Autodesk Fusion 360 part; units mm, degrees
note: some values were not read from the file. Set by a fixed rule: the direction of a hole.
(part 4 of 8)
  spline S367 degree 3 poles (-140.5026, -58.4189) (-140.4982, -58.6928) (-140.4948, -58.9667) (-140.4926, -59.2407) knots 0 0 0 0 1 1 1 1
  spline S368 degree 3 poles (-140.4926, -59.2407) (-140.4892, -59.6344) (-140.4818, -60.028) (-140.4736, -60.4216) knots 0 0 0 0 1 1 1 1
  spline S369 degree 3 poles (-140.4736, -60.4216) (-140.4734, -60.5442) (-140.4732, -60.6668) (-140.473, -60.793) knots 0 0 0 0 1 1 1 1
  spline S370 degree 3 poles (-140.473, -60.793) (-140.4555, -61.482) (-140.4555, -61.482) (-140.0812, -62.0375) knots 0 0 0 0 1 1 1 1
  spline S371 degree 3 poles (-140.0812, -62.0375) (-139.5767, -62.271) (-139.3177, -62.2016) (-138.7893, -62.0358) knots 0 0 0 0 1 1 1 1
  spline S372 degree 3 poles (-138.7893, -62.0358) (-138.1237, -61.7626) (-138.1237, -61.7626) (-137.6781, -61.2421) knots 0 0 0 0 1 1 1 1
  spline S373 degree 3 poles (-137.6781, -61.2421) (-137.5109, -60.3536) (-137.5224, -59.4745) (-137.5293, -58.5731) knots 0 0 0 0 1 1 1 1
  spline S374 degree 3 poles (-137.5293, -58.5731) (-137.5272, -58.3243) (-137.5246, -58.0755) (-137.5215, -57.8268) knots 0 0 0 0 1 1 1 1
  spline S375 degree 3 poles (-137.5215, -57.8268) (-137.515, -57.2188) (-137.5154, -56.6113) (-137.5193, -56.0033) knots 0 0 0 0 1 1 1 1
  spline S376 degree 3 poles (-137.5193, -56.0033) (-137.205, -56.0033) (-136.8907, -56.0033) (-136.5668, -56.0033) knots 0 0 0 0 1 1 1 1
  spline S377 degree 3 poles (-136.5668, -56.0033) (-136.5668, -58.256) (-136.5668, -60.5086) (-136.5668, -62.8296) knots 0 0 0 0 1 1 1 1
  spline S378 degree 3 poles (-136.5668, -62.8296) (-136.8812, -62.8296) (-137.1955, -62.8296) (-137.5193, -62.8296) knots 0 0 0 0 1 1 1 1
  spline S379 degree 3 poles (-137.5193, -62.8296) (-137.5717, -62.6724) (-137.6241, -62.5152) (-137.6781, -62.3533) knots 0 0 0 0 1 1 1 1
  spline S380 degree 3 poles (-137.6781, -62.3533) (-137.8287, -62.4581) (-137.9793, -62.5629) (-138.1345, -62.6708) knots 0 0 0 0 1 1 1 1
  spline S381 degree 3 poles (-138.1345, -62.6708) (-138.8626, -63.0806) (-139.5601, -63.1684) (-140.3768, -62.9883) knots 0 0 0 0 1 1 1 1
  spline S382 degree 3 poles (-135.0686, -77.4941) (-135.9231, -76.9719) (-136.4768, -76.235) (-136.7944, -75.284) knots 0 0 0 0 1 1 1 1
  spline S383 degree 3 poles (-136.7944, -75.284) (-137.183, -73.601) (-137.2588, -71.5992) (-136.3684, -70.0626) knots 0 0 0 0 1 1 1 1
  spline S384 degree 3 poles (-136.3684, -70.0626) (-135.7688, -69.2218) (-135.1227, -68.6286) (-134.0696, -68.4212) knots 0 0 0 0 1 1 1 1
  spline S385 degree 3 poles (-134.0696, -68.4212) (-132.935, -68.3098) (-131.9094, -68.415) (-130.9659, -69.0878) knots 0 0 0 0 1 1 1 1
  spline S386 degree 3 poles (-130.9659, -69.0878) (-129.9714, -70.0009) (-129.6245, -71.1542) (-129.5471, -72.4674) knots 0 0 0 0 1 1 1 1
  spline S387 degree 3 poles (-129.5471, -72.4674) (-129.4973, -74.0526) (-129.5833, -75.5982) (-130.6162, -76.8833) knots 0 0 0 0 1 1 1 1
  spline S388 degree 3 poles (-130.6162, -76.8833) (-131.7464, -78.0045) (-133.6433, -78.1378) (-135.0686, -77.4941) knots 0 0 0 0 1 1 1 1
  spline S389 degree 3 poles (-131.3082, -76.1546) (-130.3984, -74.7293) (-130.3552, -73.0615) (-130.6435, -71.4318) knots 0 0 0 0 1 1 1 1
  spline S390 degree 3 poles (-130.6435, -71.4318) (-130.8576, -70.6183) (-131.2038, -69.9356) (-131.9296, -69.476) knots 0 0 0 0 1 1 1 1
  spline S391 degree 3 poles (-131.9296, -69.476) (-132.7297, -69.1221) (-133.5092, -69.0729) (-134.3443, -69.3383) knots 0 0 0 0 1 1 1 1
  spline S392 degree 3 poles (-134.3443, -69.3383) (-135.012, -69.7012) (-135.4666, -70.1853) (-135.7632, -70.8861) knots 0 0 0 0 1 1 1 1
  spline S393 degree 3 poles (-135.7632, -70.8861) (-136.1825, -72.4299) (-136.191, -74.42) (-135.4897, -75.87) knots 0 0 0 0 1 1 1 1
  spline S394 degree 3 poles (-135.4897, -75.87) (-135.1461, -76.3948) (-134.7368, -76.6827) (-134.1856, -76.9583) knots 0 0 0 0 1 1 1 1
  spline S395 degree 3 poles (-134.1856, -76.9583) (-132.9719, -77.0599) (-132.2031, -77.0231) (-131.3082, -76.1546) knots 0 0 0 0 1 1 1 1
  spline S396 degree 3 poles (-144.4448, -77.4842) (-145.1477, -76.7998) (-145.4309, -76.1732) (-145.4703, -75.1952) knots 0 0 0 0 1 1 1 1
  spline S397 degree 3 poles (-145.4703, -75.1952) (-145.4752, -74.783) (-145.4747, -74.3711) (-145.4723, -73.9588) knots 0 0 0 0 1 1 1 1
  spline S398 degree 3 poles (-145.4723, -73.9588) (-145.4721, -73.8084) (-145.4719, -73.658) (-145.4717, -73.5031) knots 0 0 0 0 1 1 1 1
  spline S399 degree 3 poles (-145.4717, -73.5031) (-145.4708, -73.0243) (-145.4688, -72.5456) (-145.4668, -72.0668) knots 0 0 0 0 1 1 1 1
  spline S400 degree 3 poles (-145.4668, -72.0668) (-145.466, -71.7416) (-145.4652, -71.4163) (-145.4646, -71.0911) knots 0 0 0 0 1 1 1 1
  spline S401 degree 3 poles (-145.4646, -71.0911) (-145.4628, -70.2952) (-145.4601, -69.4992) (-145.4568, -68.7033) knots 0 0 0 0 1 1 1 1
  spline S402 degree 3 poles (-145.4568, -68.7033) (-145.1425, -68.7033) (-144.8282, -68.7033) (-144.5043, -68.7033) knots 0 0 0 0 1 1 1 1
  spline S403 degree 3 poles (-144.5043, -68.7033) (-144.4996, -68.9747) (-144.4996, -68.9747) (-144.4948, -69.2515) knots 0 0 0 0 1 1 1 1
  spline S404 degree 3 poles (-144.4948, -69.2515) (-144.4827, -69.9273) (-144.4686, -70.603) (-144.454, -71.2787) knots 0 0 0 0 1 1 1 1
  spline S405 degree 3 poles (-144.454, -71.2787) (-144.4479, -71.5703) (-144.4424, -71.8619) (-144.4374, -72.1536) knots 0 0 0 0 1 1 1 1
  spline S406 degree 3 poles (-144.4374, -72.1536) (-144.4301, -72.5745) (-144.4209, -72.9953) (-144.4113, -73.4162) knots 0 0 0 0 1 1 1 1
  spline S407 degree 3 poles (-144.4113, -73.4162) (-144.4095, -73.5451) (-144.4077, -73.6739) (-144.4058, -73.8067) knots 0 0 0 0 1 1 1 1
  spline S408 degree 3 poles (-144.4058, -73.8067) (-144.3812, -74.7731) (-144.2975, -75.7155) (-143.79, -76.5614) knots 0 0 0 0 1 1 1 1
  spline S409 degree 3 poles (-143.79, -76.5614) (-143.1421, -76.9502) (-142.5381, -76.9433) (-141.8056, -76.7996) knots 0 0 0 0 1 1 1 1
  spline S410 degree 3 poles (-141.8056, -76.7996) (-141.2743, -76.5434) (-140.8258, -76.2279) (-140.3768, -75.8471) knots 0 0 0 0 1 1 1 1
  spline S411 degree 3 poles (-140.3768, -75.8471) (-140.2675, -75.7674) (-140.1581, -75.6877) (-140.0455, -75.6055) knots 0 0 0 0 1 1 1 1
  spline S412 degree 3 poles (-140.0455, -75.6055) (-139.5872, -75.0116) (-139.6461, -74.4576) (-139.6451, -73.7263) knots 0 0 0 0 1 1 1 1
  spline S413 degree 3 poles (-139.6451, -73.7263) (-139.6425, -73.5827) (-139.6399, -73.4391) (-139.6371, -73.2912) knots 0 0 0 0 1 1 1 1
  spline S414 degree 3 poles (-139.6371, -73.2912) (-139.6294, -72.8335) (-139.6261, -72.3758) (-139.6228, -71.918) knots 0 0 0 0 1 1 1 1
  spline S415 degree 3 poles (-139.6228, -71.918) (-139.6183, -71.6073) (-139.6136, -71.2966) (-139.6085, -70.986) knots 0 0 0 0 1 1 1 1
  spline S416 degree 3 poles (-139.6085, -70.986) (-139.5968, -70.2251) (-139.5889, -69.4643) (-139.5831, -68.7033) knots 0 0 0 0 1 1 1 1
  spline S417 degree 3 poles (-139.5831, -68.7033) (-139.2688, -68.7033) (-138.9544, -68.7033) (-138.6306, -68.7033) knots 0 0 0 0 1 1 1 1
  spline S418 degree 3 poles (-138.6306, -68.7033) (-138.6306, -71.637) (-138.6306, -74.5707) (-138.6306, -77.5933) knots 0 0 0 0 1 1 1 1
  spline S419 degree 3 poles (-138.6306, -77.5933) (-138.9449, -77.5933) (-139.2592, -77.5933) (-139.5831, -77.5933) knots 0 0 0 0 1 1 1 1
  spline S420 degree 3 poles (-139.5831, -77.5933) (-139.6355, -77.1742) (-139.6879, -76.7551) (-139.7418, -76.3233) knots 0 0 0 0 1 1 1 1
  spline S421 degree 3 poles (-139.7418, -76.3233) (-139.8243, -76.3998) (-139.9068, -76.4764) (-139.9917, -76.5552) knots 0 0 0 0 1 1 1 1
  spline S422 degree 3 poles (-139.9917, -76.5552) (-140.1578, -76.7056) (-140.1578, -76.7056) (-140.3272, -76.8591) knots 0 0 0 0 1 1 1 1
  spline S423 degree 3 poles (-140.3272, -76.8591) (-140.4359, -76.9586) (-140.5446, -77.058) (-140.6565, -77.1605) knots 0 0 0 0 1 1 1 1
  spline S424 degree 3 poles (-140.6565, -77.1605) (-141.72, -77.9808) (-143.247, -78.0418) (-144.4448, -77.4842) knots 0 0 0 0 1 1 1 1
  spline S425 degree 3 poles (-91.5314, -65.4688) (-92.3003, -65.0281) (-92.7312, -64.2638) (-93.0693, -63.4646) knots 0 0 0 0 1 1 1 1
  spline S426 degree 3 poles (-93.0693, -63.4646) (-93.0693, -63.255) (-93.0693, -63.0455) (-93.0693, -62.8296) knots 0 0 0 0 1 1 1 1
  spline S427 degree 3 poles (-93.0693, -62.8296) (-92.5979, -62.751) (-92.5979, -62.751) (-92.1168, -62.6708) knots 0 0 0 0 1 1 1 1
  spline S428 degree 3 poles (-92.1168, -62.6708) (-92.0706, -62.7799) (-92.0243, -62.889) (-91.9767, -63.0013) knots 0 0 0 0 1 1 1 1
  spline S429 degree 3 poles (-91.9767, -63.0013) (-91.5673, -63.9044) (-91.5673, -63.9044) (-90.8865, -64.6056) knots 0 0 0 0 1 1 1 1
  spline S430 degree 3 poles (-90.8865, -64.6056) (-90.1962, -64.7782) (-89.6256, -64.7818) (-88.9418, -64.5758) knots 0 0 0 0 1 1 1 1
  spline S431 degree 3 poles (-88.9418, -64.5758) (-88.1429, -63.9679) (-87.7178, -63.1685) (-87.5131, -62.1946) knots 0 0 0 0 1 1 1 1
  spline S432 degree 3 poles (-87.5131, -62.1946) (-87.3782, -60.5502) (-87.2759, -58.7681) (-88.3763, -57.442) knots 0 0 0 0 1 1 1 1
  spline S433 degree 3 poles (-88.3763, -57.442) (-89.0489, -56.9006) (-89.4736, -56.7168) (-90.3675, -56.7499) knots 0 0 0 0 1 1 1 1
  spline S434 degree 3 poles (-90.3675, -56.7499) (-90.9419, -56.8344) (-91.2177, -57.0374) (-91.6406, -57.4321) knots 0 0 0 0 1 1 1 1
  spline S435 degree 3 poles (-91.6406, -57.4321) (-91.9453, -57.945) (-92.1982, -58.472) (-92.4343, -59.0196) knots 0 0 0 0 1 1 1 1
  spline S436 degree 3 poles (-92.4343, -59.0196) (-92.9058, -58.941) (-92.9058, -58.941) (-93.3868, -58.8608) knots 0 0 0 0 1 1 1 1
  spline S437 degree 3 poles (-93.3868, -58.8608) (-93.0781, -57.5907) (-92.7893, -56.7325) (-91.6307, -56.0232) knots 0 0 0 0 1 1 1 1
  spline S438 degree 3 poles (-91.6307, -56.0232) (-90.6126, -55.6519) (-89.3848, -55.655) (-88.3961, -56.1025) knots 0 0 0 0 1 1 1 1
  spline S439 degree 3 poles (-88.3961, -56.1025) (-87.2594, -56.7803) (-86.7771, -57.7907) (-86.4018, -59.0196) knots 0 0 0 0 1 1 1 1
  spline S440 degree 3 poles (-86.4018, -59.0196) (-86.3151, -59.5983) (-86.3032, -60.1614) (-86.3125, -60.746) knots 0 0 0 0 1 1 1 1
  spline S441 degree 3 poles (-86.3125, -60.746) (-86.3142, -60.8986) (-86.3158, -61.0513) (-86.3175, -61.2086) knots 0 0 0 0 1 1 1 1
  spline S442 degree 3 poles (-86.3175, -61.2086) (-86.3573, -62.5433) (-86.5695, -63.6954) (-87.4678, -64.7308) knots 0 0 0 0 1 1 1 1
  spline S443 degree 3 poles (-87.4678, -64.7308) (-88.5867, -65.7641) (-90.1023, -66.0514) (-91.5314, -65.4688) knots 0 0 0 0 1 1 1 1
  spline S444 degree 3 poles (-75.2199, -77.4246) (-75.8077, -76.9787) (-76.1975, -76.489) (-76.5593, -75.8471) knots 0 0 0 0 1 1 1 1
  spline S445 degree 3 poles (-76.5593, -75.8471) (-76.4992, -75.4955) (-76.4992, -75.4955) (-76.4006, -75.2121) knots 0 0 0 0 1 1 1 1
  spline S446 degree 3 poles (-76.4006, -75.2121) (-76.0434, -75.1525) (-76.0434, -75.1525) (-75.6068, -75.2121) knots 0 0 0 0 1 1 1 1
  spline S447 degree 3 poles (-75.6068, -75.2121) (-75.2893, -75.6486) (-75.2893, -75.6486) (-74.9718, -76.1646) knots 0 0 0 0 1 1 1 1
  spline S448 degree 3 poles (-74.9718, -76.1646) (-74.5968, -76.5964) (-74.3407, -76.7752) (-73.7725, -76.8603) knots 0 0 0 0 1 1 1 1
  spline S449 degree 3 poles (-73.7725, -76.8603) (-73.0478, -76.8898) (-72.5476, -76.8543) (-71.8861, -76.5416) knots 0 0 0 0 1 1 1 1
  spline S450 degree 3 poles (-71.8861, -76.5416) (-71.0491, -75.7658) (-70.7185, -75.0961) (-70.6478, -73.9805) knots 0 0 0 0 1 1 1 1
  spline S451 degree 3 poles (-70.6478, -73.9805) (-70.6145, -72.6646) (-70.5865, -71.4421) (-71.3206, -70.2908) knots 0 0 0 0 1 1 1 1
  spline S452 degree 3 poles (-71.3206, -70.2908) (-71.865, -69.7325) (-72.4443, -69.3461) (-73.2423, -69.3327) knots 0 0 0 0 1 1 1 1
  spline S453 degree 3 poles (-73.2423, -69.3327) (-74.082, -69.3904) (-74.6368, -69.5706) (-75.2893, -70.1321) knots 0 0 0 0 1 1 1 1
  spline S454 degree 3 poles (-75.2893, -70.1321) (-75.531, -70.4399) (-75.7244, -70.7462) (-75.9243, -71.0846) knots 0 0 0 0 1 1 1 1
  spline S455 degree 3 poles (-75.9243, -71.0846) (-76.3113, -71.025) (-76.3113, -71.025) (-76.7181, -70.9258) knots 0 0 0 0 1 1 1 1
  spline S456 degree 3 poles (-76.7181, -70.9258) (-76.7705, -70.821) (-76.8229, -70.7163) (-76.8768, -70.6083) knots 0 0 0 0 1 1 1 1
  spline S457 degree 3 poles (-76.8768, -70.6083) (-76.1895, -69.5591) (-75.4988, -68.7484) (-74.2407, -68.4447) knots 0 0 0 0 1 1 1 1
  spline S458 degree 3 poles (-74.2407, -68.4447) (-73.0035, -68.2789) (-71.9529, -68.4967) (-70.8741, -69.12) knots 0 0 0 0 1 1 1 1
  spline S459 degree 3 poles (-70.8741, -69.12) (-69.6346, -70.4658) (-69.3727, -72.0661) (-69.4348, -73.8633) knots 0 0 0 0 1 1 1 1
  spline S460 degree 3 poles (-69.4348, -73.8633) (-69.5861, -75.1844) (-69.9622, -76.3706) (-71.0229, -77.2324) knots 0 0 0 0 1 1 1 1
  spline S461 degree 3 poles (-71.0229, -77.2324) (-72.2483, -77.9539) (-73.9518, -78.1462) (-75.2199, -77.4246) knots 0 0 0 0 1 1 1 1
  spline S462 degree 3 poles (-81.9469, -77.8017) (-82.229, -77.8057) (-82.229, -77.8057) (-82.5168, -77.8097) knots 0 0 0 0 1 1 1 1
  spline S463 degree 3 poles (-82.5168, -77.8097) (-83.5585, -77.7008) (-84.1386, -77.2307) (-84.7734, -76.448) knots 0 0 0 0 1 1 1 1
  spline S464 degree 3 poles (-84.7734, -76.448) (-85.0136, -76.107) (-85.1697, -75.7696) (-85.2906, -75.3708) knots 0 0 0 0 1 1 1 1
  spline S465 degree 3 poles (-85.2906, -75.3708) (-84.9239, -75.3184) (-84.5572, -75.266) (-84.1793, -75.2121) knots 0 0 0 0 1 1 1 1
  spline S466 degree 3 poles (-84.1793, -75.2121) (-84.0909, -75.3856) (-84.0025, -75.5591) (-83.9114, -75.7379) knots 0 0 0 0 1 1 1 1
  spline S467 degree 3 poles (-83.9114, -75.7379) (-83.5902, -76.2851) (-83.3665, -76.5768) (-82.7506, -76.7996) knots 0 0 0 0 1 1 1 1
  spline S468 degree 3 poles (-82.7506, -76.7996) (-81.9142, -76.9019) (-81.2322, -76.9031) (-80.4586, -76.5515) knots 0 0 0 0 1 1 1 1
  spline S469 degree 3 poles (-80.4586, -76.5515) (-79.618, -75.7519) (-79.298, -74.8958) (-79.2258, -73.7461) knots 0 0 0 0 1 1 1 1
  spline S470 degree 3 poles (-79.2258, -73.7461) (-79.2076, -72.3792) (-79.3071, -71.3363) (-80.0022, -70.1519) knots 0 0 0 0 1 1 1 1
  spline S471 degree 3 poles (-80.0022, -70.1519) (-80.5773, -69.6235) (-81.1854, -69.3596) (-81.9705, -69.3228) knots 0 0 0 0 1 1 1 1
  spline S472 degree 3 poles (-81.9705, -69.3228) (-82.865, -69.3931) (-83.4923, -69.7332) (-84.0969, -70.3857) knots 0 0 0 0 1 1 1 1
  spline S473 degree 3 poles (-84.0969, -70.3857) (-84.2892, -70.6136) (-84.4732, -70.8486) (-84.6556, -71.0846) knots 0 0 0 0 1 1 1 1
  spline S474 degree 3 poles (-84.6556, -71.0846) (-84.9175, -70.9798) (-85.1795, -70.875) (-85.4493, -70.7671) knots 0 0 0 0 1 1 1 1
  spline S475 degree 3 poles (-85.4493, -70.7671) (-85.2327, -69.8733) (-84.5863, -69.3692) (-83.8618, -68.8621) knots 0 0 0 0 1 1 1 1
  spline S476 degree 3 poles (-83.8618, -68.8621) (-82.8383, -68.3129) (-81.8066, -68.2779) (-80.6868, -68.5446) knots 0 0 0 0 1 1 1 1
  spline S477 degree 3 poles (-80.6868, -68.5446) (-79.6942, -68.9433) (-78.9721, -69.6736) (-78.4643, -70.6083) knots 0 0 0 0 1 1 1 1
  spline S478 degree 3 poles (-78.4643, -70.6083) (-77.8857, -72.2371) (-77.869, -74.3658) (-78.5592, -75.9624) knots 0 0 0 0 1 1 1 1
  spline S479 degree 3 poles (-78.5592, -75.9624) (-79.3538, -77.2505) (-80.4628, -77.7968) (-81.9469, -77.8017) knots 0 0 0 0 1 1 1 1
  spline S480 degree 3 poles (-54.3343, -66.1633) (-54.5439, -66.1633) (-54.7534, -66.1633) (-54.9693, -66.1633) knots 0 0 0 0 1 1 1 1
  spline S481 degree 3 poles (-54.9693, -66.1633) (-55.0326, -65.9681) (-55.0326, -65.9681) (-55.0971, -65.7689) knots 0 0 0 0 1 1 1 1
  spline S482 degree 3 poles (-55.0971, -65.7689) (-55.1532, -65.5978) (-55.2092, -65.4268) (-55.267, -65.2505) knots 0 0 0 0 1 1 1 1
  spline S483 degree 3 poles (-55.267, -65.2505) (-55.3222, -65.0811) (-55.3775, -64.9116) (-55.4344, -64.737) knots 0 0 0 0 1 1 1 1
  spline S484 degree 3 poles (-55.4344, -64.737) (-55.6732, -63.9792) (-55.6732, -63.9792) (-56.2096, -63.4447) knots 0 0 0 0 1 1 1 1
  spline S485 degree 3 poles (-56.2096, -63.4447) (-56.3815, -63.376) (-56.3815, -63.376) (-56.5568, -63.3058) knots 0 0 0 0 1 1 1 1
  spline S486 degree 3 poles (-56.5568, -63.3058) (-56.678, -63.2502) (-56.7991, -63.1945) (-56.9239, -63.1371) knots 0 0 0 0 1 1 1 1
  spline S487 degree 3 poles (-56.9239, -63.1371) (-57.4326, -62.9597) (-57.9289, -62.9002) (-58.4618, -62.8296) knots 0 0 0 0 1 1 1 1
  spline S488 degree 3 poles (-58.4618, -62.8296) (-58.7175, -61.2413) (-58.8589, -59.6722) (-58.9381, -58.0671) knots 0 0 0 0 1 1 1 1
  spline S489 degree 3 poles (-58.9381, -58.0671) (-58.4142, -58.0671) (-57.8903, -58.0671) (-57.3506, -58.0671) knots 0 0 0 0 1 1 1 1
  spline S490 degree 3 poles (-57.3506, -58.0671) (-57.4554, -59.3768) (-57.5601, -60.6864) (-57.6681, -62.0358) knots 0 0 0 0 1 1 1 1
  spline S491 degree 3 poles (-57.6681, -62.0358) (-57.1966, -62.193) (-56.7251, -62.3501) (-56.2393, -62.5121) knots 0 0 0 0 1 1 1 1
  spline S492 degree 3 poles (-56.2393, -62.5121) (-55.8387, -62.7738) (-55.8387, -62.7738) (-55.5448, -63.0478) knots 0 0 0 0 1 1 1 1
  spline S493 degree 3 poles (-55.5448, -63.0478) (-55.4454, -63.1375) (-55.3459, -63.2271) (-55.2434, -63.3195) knots 0 0 0 0 1 1 1 1
  spline S494 degree 3 poles (-55.2434, -63.3195) (-54.9361, -63.6602) (-54.7243, -64.0218) (-54.4931, -64.4171) knots 0 0 0 0 1 1 1 1
  spline S495 degree 3 poles (-54.4931, -64.4171) (-54.3829, -64.376) (-54.2727, -64.3349) (-54.1592, -64.2926) knots 0 0 0 0 1 1 1 1
  spline S496 degree 3 poles (-54.1592, -64.2926) (-53.1157, -63.904) (-52.0719, -63.5163) (-51.0277, -63.1295) knots 0 0 0 0 1 1 1 1
  spline S497 degree 3 poles (-51.0277, -63.1295) (-50.491, -62.9307) (-49.9544, -62.7316) (-49.4182, -62.5316) knots 0 0 0 0 1 1 1 1
  spline S498 degree 3 poles (-49.4182, -62.5316) (-48.8997, -62.3383) (-48.3809, -62.1459) (-47.8618, -61.9542) knots 0 0 0 0 1 1 1 1
  spline S499 degree 3 poles (-47.8618, -61.9542) (-47.5696, -61.8459) (-47.2777, -61.7368) (-46.9858, -61.6276) knots 0 0 0 0 1 1 1 1
  spline S500 degree 3 poles (-46.9858, -61.6276) (-46.0012, -61.2647) (-45.0467, -60.9629) (-44.0156, -60.7658) knots 0 0 0 0 1 1 1 1
  spline S501 degree 3 poles (-44.0156, -60.7658) (-43.9632, -60.9754) (-43.9108, -61.1849) (-43.8568, -61.4008) knots 0 0 0 0 1 1 1 1
  spline S502 degree 3 poles (-43.8568, -61.4008) (-47.2803, -62.7164) (-50.7229, -63.9742) (-54.1756, -65.2108) knots 0 0 0 0 1 1 1 1
  spline S503 degree 3 poles (-54.1756, -65.2108) (-54.228, -65.5251) (-54.2804, -65.8395) (-54.3343, -66.1633) knots 0 0 0 0 1 1 1 1
  spline S504 degree 3 poles (-98.1816, -62.8854) (-98.9995, -62.4693) (-99.3887, -61.8128) (-99.6711, -60.9618) knots 0 0 0 0 1 1 1 1
  spline S505 degree 3 poles (-99.6711, -60.9618) (-99.9157, -59.6419) (-99.9009, -58.1482) (-99.2606, -56.9558) knots 0 0 0 0 1 1 1 1
  spline S506 degree 3 poles (-99.2606, -56.9558) (-98.7122, -56.309) (-98.2441, -55.8946) (-97.3922, -55.7912) knots 0 0 0 0 1 1 1 1
  spline S507 degree 3 poles (-97.3922, -55.7912) (-96.3348, -55.7777) (-95.6491, -55.8023) (-94.8156, -56.4796) knots 0 0 0 0 1 1 1 1
  spline S508 degree 3 poles (-94.8156, -56.4796) (-93.877, -57.7205) (-93.913, -59.1188) (-94.0218, -60.6071) knots 0 0 0 0 1 1 1 1
  spline S509 degree 3 poles (-94.0218, -60.6071) (-94.2128, -61.4216) (-94.4703, -62.008) (-95.0636, -62.6014) knots 0 0 0 0 1 1 1 1
  spline S510 degree 3 poles (-95.0636, -62.6014) (-95.9785, -63.1409) (-97.1673, -63.1839) (-98.1816, -62.8854) knots 0 0 0 0 1 1 1 1
  spline S511 degree 3 poles (-95.6093, -61.8771) (-94.8213, -61.0075) (-94.9108, -59.9637) (-94.9285, -58.8577) knots 0 0 0 0 1 1 1 1
  spline S512 degree 3 poles (-94.9285, -58.8577) (-94.9874, -58.0454) (-95.1459, -57.6179) (-95.6093, -56.9558) knots 0 0 0 0 1 1 1 1
  spline S513 degree 3 poles (-95.6093, -56.9558) (-96.282, -56.5074) (-96.8833, -56.5147) (-97.6731, -56.6383) knots 0 0 0 0 1 1 1 1
  spline S514 degree 3 poles (-97.6731, -56.6383) (-98.2867, -57.0857) (-98.558, -57.5121) (-98.7843, -58.2258) knots 0 0 0 0 1 1 1 1
  spline S515 degree 3 poles (-98.7843, -58.2258) (-98.8184, -58.6534) (-98.8359, -59.059) (-98.8339, -59.4859) knots 0 0 0 0 1 1 1 1
  spline S516 degree 3 poles (-98.8339, -59.4859) (-98.8365, -59.5955) (-98.8391, -59.7051) (-98.8417, -59.818) knots 0 0 0 0 1 1 1 1
  spline S517 degree 3 poles (-98.8417, -59.818) (-98.8425, -60.7013) (-98.6497, -61.3645) (-98.0303, -62.006) knots 0 0 0 0 1 1 1 1
  spline S518 degree 3 poles (-98.0303, -62.006) (-97.1344, -62.4789) (-96.4443, -62.4274) (-95.6093, -61.8771) knots 0 0 0 0 1 1 1 1
  spline S519 degree 3 poles (-117.3581, -62.7403) (-118.1286, -62.1142) (-118.4751, -61.4339) (-118.6281, -60.4483) knots 0 0 0 0 1 1 1 1
  spline S520 degree 3 poles (-118.6281, -60.4483) (-118.7082, -59.2589) (-118.7655, -58.0185) (-118.1518, -56.9558) knots 0 0 0 0 1 1 1 1
  spline S521 degree 3 poles (-118.1518, -56.9558) (-117.585, -56.322) (-117.0459, -55.899) (-116.1805, -55.8012) knots 0 0 0 0 1 1 1 1
  spline S522 degree 3 poles (-116.1805, -55.8012) (-115.2654, -55.7676) (-114.5633, -55.8098) (-113.8116, -56.3655) knots 0 0 0 0 1 1 1 1
  spline S523 degree 3 poles (-113.8116, -56.3655) (-112.9765, -57.23) (-112.8725, -58.2773) (-112.8436, -59.4363) knots 0 0 0 0 1 1 1 1
  spline S524 degree 3 poles (-112.8436, -59.4363) (-112.8811, -60.7184) (-113.0844, -61.7309) (-114.0243, -62.6708) knots 0 0 0 0 1 1 1 1
  spline S525 degree 3 poles (-114.0243, -62.6708) (-115.0204, -63.1585) (-116.3486, -63.2494) (-117.3581, -62.7403) knots 0 0 0 0 1 1 1 1
  spline S526 degree 3 poles (-114.5006, -61.8771) (-113.8043, -61.1264) (-113.7713, -60.1626) (-113.7068, -59.1783) knots 0 0 0 0 1 1 1 1
  spline S527 degree 3 poles (-113.7068, -59.1783) (-113.7675, -58.2212) (-113.9513, -57.483) (-114.6593, -56.7971) knots 0 0 0 0 1 1 1 1
  spline S528 degree 3 poles (-114.6593, -56.7971) (-115.2502, -56.5016) (-115.921, -56.5481) (-116.5643, -56.6383) knots 0 0 0 0 1 1 1 1
  spline S529 degree 3 poles (-116.5643, -56.6383) (-117.1787, -57.0863) (-117.4453, -57.5131) (-117.6756, -58.2258) knots 0 0 0 0 1 1 1 1
  spline S530 degree 3 poles (-117.6756, -58.2258) (-117.7867, -59.3795) (-117.8686, -60.6255) (-117.2427, -61.6464) knots 0 0 0 0 1 1 1 1
  spline S531 degree 3 poles (-117.2427, -61.6464) (-116.9074, -62.029) (-116.565, -62.1943) (-116.0881, -62.3533) knots 0 0 0 0 1 1 1 1
  spline S532 degree 3 poles (-116.0881, -62.3533) (-115.3872, -62.3533) (-115.0947, -62.231) (-114.5006, -61.8771) knots 0 0 0 0 1 1 1 1
  spline S533 degree 3 poles (-122.2793, -80.6096) (-122.5937, -80.6096) (-122.908, -80.6096) (-123.2318, -80.6096) knots 0 0 0 0 1 1 1 1
  spline S534 degree 3 poles (-123.2318, -80.6096) (-123.2318, -79.6142) (-123.2318, -78.6188) (-123.2318, -77.5933) knots 0 0 0 0 1 1 1 1
  spline S535 degree 3 poles (-123.2318, -77.5933) (-123.9129, -77.5933) (-124.5939, -77.5933) (-125.2956, -77.5933) knots 0 0 0 0 1 1 1 1
  spline S536 degree 3 poles (-125.2956, -77.5933) (-125.2956, -77.3314) (-125.2956, -77.0694) (-125.2956, -76.7996) knots 0 0 0 0 1 1 1 1
  spline S537 degree 3 poles (-125.2956, -76.7996) (-124.6146, -76.7996) (-123.9335, -76.7996) (-123.2318, -76.7996) knots 0 0 0 0 1 1 1 1
  spline S538 degree 3 poles (-123.2318, -76.7996) (-123.2506, -75.8361) (-123.2703, -74.8727) (-123.2909, -73.9092) knots 0 0 0 0 1 1 1 1
  spline S539 degree 3 poles (-123.2909, -73.9092) (-123.2978, -73.5814) (-123.3044, -73.2536) (-123.3108, -72.9257) knots 0 0 0 0 1 1 1 1
  spline S540 degree 3 poles (-123.3108, -72.9257) (-123.32, -72.4548) (-123.3301, -71.9839) (-123.3404, -71.5131) knots 0 0 0 0 1 1 1 1
  spline S541 degree 3 poles (-123.3404, -71.5131) (-123.343, -71.3662) (-123.3457, -71.2194) (-123.3484, -71.068) knots 0 0 0 0 1 1 1 1
  spline S542 degree 3 poles (-123.3484, -71.068) (-123.3516, -70.9314) (-123.3547, -70.7948) (-123.358, -70.654) knots 0 0 0 0 1 1 1 1
  spline S543 degree 3 poles (-123.358, -70.654) (-123.3605, -70.5338) (-123.3629, -70.4136) (-123.3655, -70.2897) knots 0 0 0 0 1 1 1 1
  spline S544 degree 3 poles (-123.3655, -70.2897) (-123.3805, -69.9401) (-123.3805, -69.9401) (-123.5493, -69.4971) knots 0 0 0 0 1 1 1 1
  spline S545 degree 3 poles (-123.5493, -69.4971) (-124.1406, -69.3871) (-124.6941, -69.3206) (-125.2956, -69.3383) knots 0 0 0 0 1 1 1 1
  spline S546 degree 3 poles (-125.2956, -69.3383) (-125.2956, -69.0764) (-125.2956, -68.8144) (-125.2956, -68.5446) knots 0 0 0 0 1 1 1 1
  spline S547 degree 3 poles (-125.2956, -68.5446) (-124.2448, -68.3691) (-123.5325, -68.3162) (-122.5968, -68.8621) knots 0 0 0 0 1 1 1 1
  spline S548 degree 3 poles (-122.5968, -68.8621) (-122.2581, -69.3701) (-122.2402, -69.4949) (-122.2433, -70.0773) knots 0 0 0 0 1 1 1 1
  spline S549 degree 3 poles (-122.2433, -70.0773) (-122.2433, -70.2266) (-122.2433, -70.376) (-122.2434, -70.5299) knots 0 0 0 0 1 1 1 1
  spline S550 degree 3 poles (-122.2434, -70.5299) (-122.245, -70.6906) (-122.2466, -70.8514) (-122.2483, -71.017) knots 0 0 0 0 1 1 1 1
  spline S551 degree 3 poles (-122.2483, -71.017) (-122.2488, -71.1819) (-122.2492, -71.3468) (-122.2497, -71.5168) knots 0 0 0 0 1 1 1 1
  spline S552 degree 3 poles (-122.2497, -71.5168) (-122.2515, -72.0441) (-122.2555, -72.5714) (-122.2595, -73.0987) knots 0 0 0 0 1 1 1 1
  spline S553 degree 3 poles (-122.2595, -73.0987) (-122.2611, -73.456) (-122.2625, -73.8133) (-122.2638, -74.1706) knots 0 0 0 0 1 1 1 1
  spline S554 degree 3 poles (-122.2638, -74.1706) (-122.2673, -75.0469) (-122.2727, -75.9232) (-122.2793, -76.7996) knots 0 0 0 0 1 1 1 1
  spline S555 degree 3 poles (-122.2793, -76.7996) (-121.8602, -76.7996) (-121.4411, -76.7996) (-121.0093, -76.7996) knots 0 0 0 0 1 1 1 1
  spline S556 degree 3 poles (-121.0093, -76.7996) (-121.0093, -77.0615) (-121.0093, -77.3234) (-121.0093, -77.5933) knots 0 0 0 0 1 1 1 1
  spline S557 degree 3 poles (-121.0093, -77.5933) (-121.4284, -77.5933) (-121.8475, -77.5933) (-122.2793, -77.5933) knots 0 0 0 0 1 1 1 1
  spline S558 degree 3 poles (-122.2793, -77.5933) (-122.2793, -78.5887) (-122.2793, -79.584) (-122.2793, -80.6096) knots 0 0 0 0 1 1 1 1
  spline S559 degree 3 poles (-129.8993, -62.8296) (-130.2137, -62.8296) (-130.528, -62.8296) (-130.8518, -62.8296) knots 0 0 0 0 1 1 1 1
  spline S560 degree 3 poles (-130.8518, -62.8296) (-130.8542, -62.675) (-130.8565, -62.5205) (-130.8589, -62.3613) knots 0 0 0 0 1 1 1 1
  spline S561 degree 3 poles (-130.8589, -62.3613) (-130.8681, -61.7858) (-130.8803, -61.2104) (-130.8935, -60.6349) knots 0 0 0 0 1 1 1 1
  spline S562 degree 3 poles (-130.8935, -60.6349) (-130.8988, -60.3863) (-130.9032, -60.1376) (-130.9068, -59.8889) knots 0 0 0 0 1 1 1 1
  spline S563 degree 3 poles (-130.9068, -59.8889) (-130.9122, -59.5306) (-130.9205, -59.1725) (-130.9294, -58.8143) knots 0 0 0 0 1 1 1 1
  spline S564 degree 3 poles (-130.9294, -58.8143) (-130.9304, -58.7038) (-130.9314, -58.5933) (-130.9324, -58.4795) knots 0 0 0 0 1 1 1 1
  spline S565 degree 3 poles (-130.9324, -58.4795) (-130.953, -57.7919) (-131.0643, -57.3444) (-131.4868, -56.7971) knots 0 0 0 0 1 1 1 1
  spline S566 degree 3 poles (-131.4868, -56.7971) (-132.0786, -56.5881) (-132.6837, -56.7117) (-133.2624, -56.9247) knots 0 0 0 0 1 1 1 1
  spline S567 degree 3 poles (-133.2624, -56.9247) (-133.6693, -57.1655) (-133.9079, -57.3628) (-134.1856, -57.7496) knots 0 0 0 0 1 1 1 1
  spline S568 degree 3 poles (-134.1856, -57.7496) (-134.3681, -58.6167) (-134.3564, -59.4664) (-134.3443, -60.3491) knots 0 0 0 0 1 1 1 1
  spline S569 degree 3 poles (-134.3443, -60.3491) (-134.3456, -60.5895) (-134.3475, -60.8299) (-134.3499, -61.0703) knots 0 0 0 0 1 1 1 1
  spline S570 degree 3 poles (-134.3499, -61.0703) (-134.3546, -61.6568) (-134.3516, -62.243) (-134.3443, -62.8296) knots 0 0 0 0 1 1 1 1
  spline S571 degree 3 poles (-134.3443, -62.8296) (-134.6587, -62.8296) (-134.973, -62.8296) (-135.2968, -62.8296) knots 0 0 0 0 1 1 1 1
  spline S572 degree 3 poles (-135.2968, -62.8296) (-135.2968, -60.5769) (-135.2968, -58.3242) (-135.2968, -56.0033) knots 0 0 0 0 1 1 1 1
  spline S573 degree 3 poles (-135.2968, -56.0033) (-134.9825, -56.0033) (-134.6682, -56.0033) (-134.3443, -56.0033) knots 0 0 0 0 1 1 1 1
  spline S574 degree 3 poles (-134.3443, -56.0033) (-134.292, -56.2129) (-134.2396, -56.4224) (-134.1856, -56.6383) knots 0 0 0 0 1 1 1 1
  spline S575 degree 3 poles (-134.1856, -56.6383) (-134.0785, -56.5524) (-134.0785, -56.5524) (-133.9692, -56.4647) knots 0 0 0 0 1 1 1 1
  spline S576 degree 3 poles (-133.9692, -56.4647) (-133.0551, -55.8052) (-132.2815, -55.6842) (-131.1693, -55.8446) knots 0 0 0 0 1 1 1 1
  spline S577 degree 3 poles (-131.1693, -55.8446) (-130.6803, -56.0442) (-130.4727, -56.1799) (-130.1772, -56.6085) knots 0 0 0 0 1 1 1 1
  spline S578 degree 3 poles (-130.1772, -56.6085) (-129.899, -57.4198) (-129.8803, -58.227) (-129.8838, -59.0779) knots 0 0 0 0 1 1 1 1
  spline S579 degree 3 poles (-129.8838, -59.0779) (-129.8841, -59.1857) (-129.8843, -59.2936) (-129.8845, -59.4048) knots 0 0 0 0 1 1 1 1
  spline S580 degree 3 poles (-129.8845, -59.4048) (-129.8854, -59.746) (-129.8874, -60.0872) (-129.8894, -60.4285) knots 0 0 0 0 1 1 1 1
  spline S581 degree 3 poles (-129.8894, -60.4285) (-129.8902, -60.6612) (-129.8909, -60.894) (-129.8916, -61.1267) knots 0 0 0 0 1 1 1 1
  spline S582 degree 3 poles (-129.8916, -61.1267) (-129.8933, -61.6943) (-129.8961, -62.262) (-129.8993, -62.8296) knots 0 0 0 0 1 1 1 1
  spline S583 degree 3 poles (-47.9843, -59.6546) (-47.9843, -59.445) (-47.9843, -59.2355) (-47.9843, -59.0196) knots 0 0 0 0 1 1 1 1
  spline S584 degree 3 poles (-47.9843, -59.0196) (-47.7483, -58.8079) (-47.7483, -58.8079) (-47.4126, -58.619) knots 0 0 0 0 1 1 1 1
  spline S585 degree 3 poles (-47.4126, -58.619) (-47.2874, -58.5465) (-47.1621, -58.4741) (-47.0331, -58.3995) knots 0 0 0 0 1 1 1 1
  spline S586 degree 3 poles (-47.0331, -58.3995) (-46.8952, -58.3225) (-46.7572, -58.2456) (-46.6151, -58.1663) knots 0 0 0 0 1 1 1 1
  spline S587 degree 3 poles (-46.6151, -58.1663) (-46.3215, -57.9966) (-46.0282, -57.8265) (-45.7352, -57.6559) knots 0 0 0 0 1 1 1 1
  spline S588 degree 3 poles (-45.7352, -57.6559) (-45.5822, -57.5673) (-45.4293, -57.4788) (-45.2717, -57.3875) knots 0 0 0 0 1 1 1 1
  spline S589 degree 3 poles (-45.2717, -57.3875) (-44.527, -56.9479) (-43.8003, -56.481) (-43.073, -56.0132) knots 0 0 0 0 1 1 1 1
  spline S590 degree 3 poles (-43.073, -56.0132) (-41.8696, -55.2432) (-40.6638, -54.4773) (-39.4515, -53.7213) knots 0 0 0 0 1 1 1 1
  spline S591 degree 3 poles (-39.4515, -53.7213) (-39.2373, -53.5865) (-39.2373, -53.5865) (-39.0187, -53.4491) knots 0 0 0 0 1 1 1 1
  spline S592 degree 3 poles (-39.0187, -53.4491) (-38.8873, -53.3674) (-38.7559, -53.2858) (-38.6206, -53.2016) knots 0 0 0 0 1 1 1 1
  spline S593 degree 3 poles (-38.6206, -53.2016) (-38.5048, -53.1293) (-38.389, -53.057) (-38.2697, -52.9825) knots 0 0 0 0 1 1 1 1
  spline S594 degree 3 poles (-38.2697, -52.9825) (-37.9831, -52.8283) (-37.9831, -52.8283) (-37.6656, -52.8283) knots 0 0 0 0 1 1 1 1
  spline S595 degree 3 poles (-37.6656, -52.8283) (-37.154, -53.65) (-37.154, -53.65) (-37.0306, -53.9396) knots 0 0 0 0 1 1 1 1
  spline S596 degree 3 poles (-37.0306, -53.9396) (-37.2254, -54.5239) (-37.3463, -54.5438) (-37.8808, -54.8121) knots 0 0 0 0 1 1 1 1
  spline S597 degree 3 poles (-37.8808, -54.8121) (-38.027, -54.8867) (-38.1733, -54.9613) (-38.324, -55.0382) knots 0 0 0 0 1 1 1 1
  spline S598 degree 3 poles (-38.324, -55.0382) (-38.4833, -55.1177) (-38.6425, -55.1971) (-38.8066, -55.279) knots 0 0 0 0 1 1 1 1
  spline S599 degree 3 poles (-38.8066, -55.279) (-39.1422, -55.4501) (-39.4777, -55.6214) (-39.8131, -55.7931) knots 0 0 0 0 1 1 1 1
  spline S600 degree 3 poles (-39.8131, -55.7931) (-39.9845, -55.8806) (-40.156, -55.9681) (-40.3326, -56.0583) knots 0 0 0 0 1 1 1 1
  spline S601 degree 3 poles (-40.3326, -56.0583) (-41.1043, -56.4571) (-41.8655, -56.8744) (-42.6265, -57.2932) knots 0 0 0 0 1 1 1 1
  spline S602 degree 3 poles (-42.6265, -57.2932) (-42.913, -57.4497) (-43.1995, -57.6062) (-43.486, -57.7626) knots 0 0 0 0 1 1 1 1
  spline S603 degree 3 poles (-43.486, -57.7626) (-43.9139, -57.9963) (-44.3414, -58.2304) (-44.7683, -58.466) knots 0 0 0 0 1 1 1 1
  spline S604 degree 3 poles (-44.7683, -58.466) (-45.1845, -58.6954) (-45.602, -58.9222) (-46.0198, -59.1485) knots 0 0 0 0 1 1 1 1
  spline S605 degree 3 poles (-46.0198, -59.1485) (-46.1449, -59.2183) (-46.27, -59.288) (-46.3989, -59.3598) knots 0 0 0 0 1 1 1 1
  spline S606 degree 3 poles (-46.3989, -59.3598) (-46.5728, -59.4532) (-46.5728, -59.4532) (-46.7503, -59.5485) knots 0 0 0 0 1 1 1 1
  spline S607 degree 3 poles (-46.7503, -59.5485) (-46.8511, -59.6037) (-46.9519, -59.659) (-47.0558, -59.7158) knots 0 0 0 0 1 1 1 1
  spline S608 degree 3 poles (-47.0558, -59.7158) (-47.4209, -59.8371) (-47.6258, -59.7774) (-47.9843, -59.6546) knots 0 0 0 0 1 1 1 1
  spline S609 degree 3 poles (-105.303, -62.7899) (-105.8326, -62.3115) (-105.9216, -61.9879) (-105.9641, -61.2658) knots 0 0 0 0 1 1 1 1
  spline S610 degree 3 poles (-105.9641, -61.2658) (-105.9641, -61.0206) (-105.9623, -60.7754) (-105.9591, -60.5302) knots 0 0 0 0 1 1 1 1
  spline S611 degree 3 poles (-105.9591, -60.5302) (-105.9586, -60.4007) (-105.9582, -60.2712) (-105.9577, -60.1378) knots 0 0 0 0 1 1 1 1
  spline S612 degree 3 poles (-105.9577, -60.1378) (-105.956, -59.7254) (-105.952, -59.3129) (-105.9479, -58.9005) knots 0 0 0 0 1 1 1 1
  spline S613 degree 3 poles (-105.9479, -58.9005) (-105.9463, -58.6204) (-105.9449, -58.3403) (-105.9436, -58.0602) knots 0 0 0 0 1 1 1 1
  spline S614 degree 3 poles (-105.9436, -58.0602) (-105.9401, -57.3746) (-105.9346, -56.689) (-105.9281, -56.0033) knots 0 0 0 0 1 1 1 1
  spline S615 degree 3 poles (-105.9281, -56.0033) (-105.6662, -56.0033) (-105.4042, -56.0033) (-105.1343, -56.0033) knots 0 0 0 0 1 1 1 1
  spline S616 degree 3 poles (-105.1343, -56.0033) (-105.1312, -56.153) (-105.128, -56.3028) (-105.1248, -56.457) knots 0 0 0 0 1 1 1 1
  spline S617 degree 3 poles (-105.1248, -56.457) (-105.1124, -57.0148) (-105.0986, -57.5724) (-105.084, -58.1301) knots 0 0 0 0 1 1 1 1
  spline S618 degree 3 poles (-105.084, -58.1301) (-105.0779, -58.3711) (-105.0724, -58.612) (-105.0674, -58.853) knots 0 0 0 0 1 1 1 1
  spline S619 degree 3 poles (-105.0674, -58.853) (-105.0601, -59.2002) (-105.0509, -59.5474) (-105.0413, -59.8946) knots 0 0 0 0 1 1 1 1
  spline S620 degree 3 poles (-105.0413, -59.8946) (-105.0363, -60.1032) (-105.0313, -60.3119) (-105.0262, -60.5269) knots 0 0 0 0 1 1 1 1
  spline S621 degree 3 poles (-105.0262, -60.5269) (-104.9786, -61.0501) (-104.896, -61.4121) (-104.6581, -61.8771) knots 0 0 0 0 1 1 1 1
  spline S622 degree 3 poles (-104.6581, -61.8771) (-104.2824, -62.1723) (-104.0645, -62.1946) (-103.5865, -62.1946) knots 0 0 0 0 1 1 1 1
  spline S623 degree 3 poles (-103.5865, -62.1946) (-102.8341, -61.9631) (-102.2812, -61.7286) (-101.8006, -61.0833) knots 0 0 0 0 1 1 1 1
  spline S624 degree 3 poles (-101.8006, -61.0833) (-101.6166, -60.2167) (-101.6298, -59.3663) (-101.6418, -58.4838) knots 0 0 0 0 1 1 1 1
  spline S625 degree 3 poles (-101.6418, -58.4838) (-101.6406, -58.2434) (-101.6387, -58.003) (-101.6363, -57.7626) knots 0 0 0 0 1 1 1 1
  spline S626 degree 3 poles (-101.6363, -57.7626) (-101.6315, -57.176) (-101.6346, -56.5898) (-101.6418, -56.0033) knots 0 0 0 0 1 1 1 1
  spline S627 degree 3 poles (-101.6418, -56.0033) (-101.3275, -56.0033) (-101.0132, -56.0033) (-100.6893, -56.0033) knots 0 0 0 0 1 1 1 1
  spline S628 degree 3 poles (-100.6893, -56.0033) (-100.6893, -58.256) (-100.6893, -60.5086) (-100.6893, -62.8296) knots 0 0 0 0 1 1 1 1
  spline S629 degree 3 poles (-100.6893, -62.8296) (-101.0037, -62.8296) (-101.318, -62.8296) (-101.6418, -62.8296) knots 0 0 0 0 1 1 1 1
  spline S630 degree 3 poles (-101.6418, -62.8296) (-101.6942, -62.62) (-101.7466, -62.4105) (-101.8006, -62.1946) knots 0 0 0 0 1 1 1 1
  spline S631 degree 3 poles (-101.8006, -62.1946) (-101.9217, -62.2961) (-102.0429, -62.3976) (-102.1677, -62.5021) knots 0 0 0 0 1 1 1 1
  spline S632 degree 3 poles (-102.1677, -62.5021) (-103.046, -63.1762) (-104.2919, -63.2026) (-105.303, -62.7899) knots 0 0 0 0 1 1 1 1
  spline S633 degree 3 poles (-110.8927, -62.8686) (-111.4222, -62.5838) (-111.7743, -62.298) (-111.9606, -61.7183) knots 0 0 0 0 1 1 1 1
  spline S634 degree 3 poles (-111.9606, -61.7183) (-111.8034, -61.5612) (-111.6463, -61.404) (-111.4843, -61.2421) knots 0 0 0 0 1 1 1 1
  spline S635 degree 3 poles (-111.4843, -61.2421) (-111.1352, -61.4042) (-110.8486, -61.5602) (-110.5517, -61.8076) knots 0 0 0 0 1 1 1 1
  spline S636 degree 3 poles (-110.5517, -61.8076) (-109.9897, -62.1878) (-109.4666, -62.2257) (-108.8054, -62.1251) knots 0 0 0 0 1 1 1 1
  spline S637 degree 3 poles (-108.8054, -62.1251) (-108.6384, -62.0809) (-108.6384, -62.0809) (-108.4681, -62.0358) knots 0 0 0 0 1 1 1 1
  spline S638 degree 3 poles (-108.4681, -62.0358) (-108.4157, -61.5643) (-108.3633, -61.0928) (-108.3093, -60.6071) knots 0 0 0 0 1 1 1 1
  spline S639 degree 3 poles (-108.3093, -60.6071) (-108.5091, -60.5416) (-108.7088, -60.4761) (-108.9146, -60.4086) knots 0 0 0 0 1 1 1 1
  spline S640 degree 3 poles (-108.9146, -60.4086) (-109.0439, -60.3648) (-109.1732, -60.321) (-109.3065, -60.2759) knots 0 0 0 0 1 1 1 1
  spline S641 degree 3 poles (-109.3065, -60.2759) (-109.6032, -60.1762) (-109.9009, -60.0796) (-110.1995, -59.9857) knots 0 0 0 0 1 1 1 1
  spline S642 degree 3 poles (-110.1995, -59.9857) (-110.8549, -59.769) (-111.3732, -59.5911) (-111.9011, -59.1386) knots 0 0 0 0 1 1 1 1
  spline S643 degree 3 poles (-111.9011, -59.1386) (-112.2866, -58.3676) (-112.3741, -57.7442) (-112.1193, -56.9161) knots 0 0 0 0 1 1 1 1
  spline S644 degree 3 poles (-112.1193, -56.9161) (-111.7195, -56.3663) (-111.3318, -56.0517) (-110.6906, -55.8446) knots 0 0 0 0 1 1 1 1
  spline S645 degree 3 poles (-110.6906, -55.8446) (-109.5701, -55.6809) (-108.5981, -55.7992) (-107.6743, -56.4796) knots 0 0 0 0 1 1 1 1
  spline S646 degree 3 poles (-107.6743, -56.4796) (-107.2775, -56.9161) (-107.2775, -56.9161) (-107.0393, -57.2733) knots 0 0 0 0 1 1 1 1
  spline S647 degree 3 poles (-107.0393, -57.2733) (-107.1965, -57.4305) (-107.3537, -57.5876) (-107.5156, -57.7496) knots 0 0 0 0 1 1 1 1
  spline S648 degree 3 poles (-107.5156, -57.7496) (-107.919, -57.5703) (-108.1718, -57.4109) (-108.4879, -57.0947) knots 0 0 0 0 1 1 1 1
  spline S649 degree 3 poles (-108.4879, -57.0947) (-109.1523, -56.6614) (-109.7595, -56.6681) (-110.5318, -56.7971) knots 0 0 0 0 1 1 1 1
  spline S650 degree 3 poles (-110.5318, -56.7971) (-111.0153, -57.1079) (-111.1312, -57.2736) (-111.2561, -57.8289) knots 0 0 0 0 1 1 1 1
  spline S651 degree 3 poles (-111.2561, -57.8289) (-111.1271, -58.4026) (-110.8546, -58.5329) (-110.3731, -58.8608) knots 0 0 0 0 1 1 1 1
  spline S652 degree 3 poles (-110.3731, -58.8608) (-109.8697, -59.0472) (-109.3709, -59.2015) (-108.8554, -59.3476) knots 0 0 0 0 1 1 1 1
  spline S653 degree 3 poles (-108.8554, -59.3476) (-108.2021, -59.5459) (-107.7646, -59.7317) (-107.3568, -60.2896) knots 0 0 0 0 1 1 1 1
  spline S654 degree 3 poles (-107.3568, -60.2896) (-107.2035, -60.9303) (-107.2092, -61.596) (-107.5193, -62.1865) knots 0 0 0 0 1 1 1 1
  spline S655 degree 3 poles (-107.5193, -62.1865) (-108.3177, -63.1857) (-109.7217, -63.257) (-110.8927, -62.8686) knots 0 0 0 0 1 1 1 1
  spline S656 degree 3 poles (-96.0856, -81.0858) (-96.4523, -81.0858) (-96.819, -81.0858) (-97.1968, -81.0858) knots 0 0 0 0 1 1 1 1
  spline S657 degree 3 poles (-97.1968, -81.0858) (-97.1968, -76.9996) (-97.1968, -72.9134) (-97.1968, -68.7033) knots 0 0 0 0 1 1 1 1
  spline S658 degree 3 poles (-97.1968, -68.7033) (-96.8301, -68.7033) (-96.4634, -68.7033) (-96.0856, -68.7033) knots 0 0 0 0 1 1 1 1
  spline S659 degree 3 poles (-96.0856, -68.7033) (-96.0856, -72.7895) (-96.0856, -76.8758) (-96.0856, -81.0858) knots 0 0 0 0 1 1 1 1
  spline S660 degree 3 poles (-53.5406, -58.7021) (-53.868, -58.6326) (-53.868, -58.6326) (-54.1756, -58.5433) knots 0 0 0 0 1 1 1 1
  spline S661 degree 3 poles (-54.1756, -58.5433) (-54.0768, -57.8575) (-53.8312, -57.3312) (-53.5127, -56.7183) knots 0 0 0 0 1 1 1 1
  spline S662 degree 3 poles (-53.5127, -56.7183) (-53.4361, -56.5702) (-53.4361, -56.5702) (-53.358, -56.4191) knots 0 0 0 0 1 1 1 1
  spline S663 degree 3 poles (-53.358, -56.4191) (-53.1917, -56.098) (-53.0239, -55.7778) (-52.856, -55.4576) knots 0 0 0 0 1 1 1 1
  spline S664 degree 3 poles (-52.856, -55.4576) (-52.7409, -55.2364) (-52.6258, -55.0152) (-52.5108, -54.7939) knots 0 0 0 0 1 1 1 1
  spline S665 degree 3 poles (-52.5108, -54.7939) (-51.6109, -53.0669) (-50.6875, -51.3531) (-49.7424, -49.6504) knots 0 0 0 0 1 1 1 1
  spline S666 degree 3 poles (-49.7424, -49.6504) (-49.5726, -49.3371) (-49.4119, -49.0205) (-49.2543, -48.7008) knots 0 0 0 0 1 1 1 1
  spline S667 degree 3 poles (-49.2543, -48.7008) (-48.7649, -48.8912) (-48.2919, -49.094) (-47.8256, -49.3358) knots 0 0 0 0 1 1 1 1
  spline S668 degree 3 poles (-47.8256, -49.3358) (-48.0735, -50.3099) (-48.6123, -51.0746) (-49.1551, -51.9056) knots 0 0 0 0 1 1 1 1
  spline S669 degree 3 poles (-49.1551, -51.9056) (-49.3567, -52.2181) (-49.5583, -52.5306) (-49.7597, -52.8432) knots 0 0 0 0 1 1 1 1
  spline S670 degree 3 poles (-49.7597, -52.8432) (-49.8612, -53) (-49.9627, -53.1567) (-50.0672, -53.3182) knots 0 0 0 0 1 1 1 1
  spline S671 degree 3 poles (-50.0672, -53.3182) (-50.5123, -54.0084) (-50.9501, -54.7031) (-51.3875, -55.3981) knots 0 0 0 0 1 1 1 1
  spline S672 degree 3 poles (-51.3875, -55.3981) (-51.5421, -55.643) (-51.6967, -55.888) (-51.8514, -56.1329) knots 0 0 0 0 1 1 1 1
  spline S673 degree 3 poles (-51.8514, -56.1329) (-52.0535, -56.4531) (-52.2555, -56.7732) (-52.4576, -57.0934) knots 0 0 0 0 1 1 1 1
  spline S674 degree 3 poles (-52.4576, -57.0934) (-52.6166, -57.3453) (-52.776, -57.5971) (-52.9354, -57.8488) knots 0 0 0 0 1 1 1 1
  spline S675 degree 3 poles (-52.9354, -57.8488) (-53.0195, -57.9818) (-53.1036, -58.1148) (-53.1902, -58.2519) knots 0 0 0 0 1 1 1 1
  spline S676 degree 3 poles (-53.1902, -58.2519) (-53.3818, -58.5433) (-53.3818, -58.5433) (-53.5406, -58.7021) knots 0 0 0 0 1 1 1 1
  spline S677 degree 3 poles (-48.6505, -56.5841) (-48.7922, -56.5324) (-48.7922, -56.5324) (-48.9368, -56.4796) knots 0 0 0 0 1 1 1 1
  spline S678 degree 3 poles (-48.9368, -56.4796) (-48.8447, -55.9731) (-48.7068, -55.714) (-48.3432, -55.3524) knots 0 0 0 0 1 1 1 1
  spline S679 degree 3 poles (-48.3432, -55.3524) (-48.2508, -55.2593) (-48.1584, -55.1663) (-48.0632, -55.0704) knots 0 0 0 0 1 1 1 1
  spline S680 degree 3 poles (-48.0632, -55.0704) (-47.9613, -54.9703) (-47.8595, -54.8701) (-47.7545, -54.767) knots 0 0 0 0 1 1 1 1
  spline S681 degree 3 poles (-47.7545, -54.767) (-47.6477, -54.66) (-47.5408, -54.5531) (-47.4307, -54.4429) knots 0 0 0 0 1 1 1 1
  spline S682 degree 3 poles (-47.4307, -54.4429) (-47.0771, -54.0896) (-46.7218, -53.738) (-46.3665, -53.3864) knots 0 0 0 0 1 1 1 1
  spline S683 degree 3 poles (-46.3665, -53.3864) (-46.121, -53.1418) (-45.8756, -52.8972) (-45.6304, -52.6524) knots 0 0 0 0 1 1 1 1
  spline S684 degree 3 poles (-45.6304, -52.6524) (-44.9844, -52.0083) (-44.3371, -51.3656) (-43.6894, -50.7232) knots 0 0 0 0 1 1 1 1
  spline S685 degree 3 poles (-43.6894, -50.7232) (-43.0289, -50.0675) (-42.3696, -49.4105) (-41.7103, -48.7535) knots 0 0 0 0 1 1 1 1
  spline S686 degree 3 poles (-41.7103, -48.7535) (-40.4163, -47.4646) (-39.1208, -46.1773) (-37.8243, -44.8908) knots 0 0 0 0 1 1 1 1
  spline S687 degree 3 poles (-37.8243, -44.8908) (-37.6148, -45.1004) (-37.4052, -45.3099) (-37.1893, -45.5258) knots 0 0 0 0 1 1 1 1
  spline S688 degree 3 poles (-37.1893, -45.5258) (-38.6249, -46.9798) (-40.0626, -48.4316) (-41.5031, -49.8807) knots 0 0 0 0 1 1 1 1
  spline S689 degree 3 poles (-41.5031, -49.8807) (-42.1719, -50.5536) (-42.8398, -51.2272) (-43.5062, -51.9025) knots 0 0 0 0 1 1 1 1
  spline S690 degree 3 poles (-43.5062, -51.9025) (-44.1488, -52.5537) (-44.7933, -53.203) (-45.4392, -53.851) knots 0 0 0 0 1 1 1 1
  spline S691 degree 3 poles (-45.4392, -53.851) (-45.6858, -54.099) (-45.9316, -54.3477) (-46.1767, -54.5971) knots 0 0 0 0 1 1 1 1
  spline S692 degree 3 poles (-46.1767, -54.5971) (-46.5192, -54.9453) (-46.8641, -55.291) (-47.2097, -55.6362) knots 0 0 0 0 1 1 1 1
  spline S693 degree 3 poles (-47.2097, -55.6362) (-47.3621, -55.793) (-47.3621, -55.793) (-47.5176, -55.9529) knots 0 0 0 0 1 1 1 1
  spline S694 degree 3 poles (-47.5176, -55.9529) (-47.612, -56.0461) (-47.7064, -56.1394) (-47.8036, -56.2355) knots 0 0 0 0 1 1 1 1
  spline S695 degree 3 poles (-47.8036, -56.2355) (-47.9256, -56.3587) (-47.9256, -56.3587) (-48.0502, -56.4843) knots 0 0 0 0 1 1 1 1
  spline S696 degree 3 poles (-48.0502, -56.4843) (-48.3018, -56.6383) (-48.3018, -56.6383) (-48.6505, -56.5841) knots 0 0 0 0 1 1 1 1
  spline S697 degree 3 poles (-112.5956, -77.7521) (-112.5956, -77.4377) (-112.5956, -77.1234) (-112.5956, -76.7996) knots 0 0 0 0 1 1 1 1
  spline S698 degree 3 poles (-112.5956, -76.7996) (-112.5035, -76.7859) (-112.4114, -76.7721) (-112.3165, -76.758) knots 0 0 0 0 1 1 1 1
  spline S699 degree 3 poles (-112.3165, -76.758) (-111.4595, -76.6039) (-110.7689, -76.4006) (-110.2143, -75.6883) knots 0 0 0 0 1 1 1 1
  spline S700 degree 3 poles (-110.2143, -75.6883) (-109.4017, -74.3273) (-109.474, -72.833) (-109.4603, -71.3028) knots 0 0 0 0 1 1 1 1
  spline S701 degree 3 poles (-109.4603, -71.3028) (-109.4558, -71.05) (-109.451, -70.7972) (-109.446, -70.5444) knots 0 0 0 0 1 1 1 1
  spline S702 degree 3 poles (-109.446, -70.5444) (-109.4344, -69.9307) (-109.4265, -69.3171) (-109.4206, -68.7033) knots 0 0 0 0 1 1 1 1
  spline S703 degree 3 poles (-109.4206, -68.7033) (-109.1063, -68.7033) (-108.7919, -68.7033) (-108.4681, -68.7033) knots 0 0 0 0 1 1 1 1
  spline S704 degree 3 poles (-108.4681, -68.7033) (-108.4681, -71.637) (-108.4681, -74.5707) (-108.4681, -77.5933) knots 0 0 0 0 1 1 1 1
  spline S705 degree 3 poles (-108.4681, -77.5933) (-108.7824, -77.5933) (-109.0967, -77.5933) (-109.4206, -77.5933) knots 0 0 0 0 1 1 1 1
  spline S706 degree 3 poles (-109.4206, -77.5933) (-109.473, -77.1218) (-109.5254, -76.6503) (-109.5793, -76.1646) knots 0 0 0 0 1 1 1 1
  spline S707 degree 3 poles (-109.5793, -76.1646) (-109.6612, -76.3086) (-109.743, -76.4527) (-109.8274, -76.6011) knots 0 0 0 0 1 1 1 1
  spline S708 degree 3 poles (-109.8274, -76.6011) (-110.5302, -77.6417) (-111.3946, -77.8363) (-112.5956, -77.7521) knots 0 0 0 0 1 1 1 1
  spline S709 degree 3 poles (-124.3431, -65.2108) (-124.6574, -65.2108) (-124.9717, -65.2108) (-125.2956, -65.2108) knots 0 0 0 0 1 1 1 1
  spline S710 degree 3 poles (-125.2956, -65.2108) (-125.2956, -64.425) (-125.2956, -63.6392) (-125.2956, -62.8296) knots 0 0 0 0 1 1 1 1
  spline S711 degree 3 poles (-125.2956, -62.8296) (-125.7671, -62.8296) (-126.2386, -62.8296) (-126.7243, -62.8296) knots 0 0 0 0 1 1 1 1
  spline S712 degree 3 poles (-126.7243, -62.8296) (-126.7243, -62.62) (-126.7243, -62.4105) (-126.7243, -62.1946) knots 0 0 0 0 1 1 1 1
  spline S713 degree 3 poles (-126.7243, -62.1946) (-126.2529, -62.1946) (-125.7814, -62.1946) (-125.2956, -62.1946) knots 0 0 0 0 1 1 1 1
  spline S714 degree 3 poles (-125.2956, -62.1946) (-125.348, -60.4134) (-125.4004, -58.6322) (-125.4543, -56.7971) knots 0 0 0 0 1 1 1 1
  spline S715 degree 3 poles (-125.4543, -56.7971) (-125.8734, -56.7447) (-126.2925, -56.6923) (-126.7243, -56.6383) knots 0 0 0 0 1 1 1 1
  spline S716 degree 3 poles (-126.7243, -56.6383) (-126.7243, -56.3764) (-126.7243, -56.1144) (-126.7243, -55.8446) knots 0 0 0 0 1 1 1 1
  spline S717 degree 3 poles (-126.7243, -55.8446) (-126.4767, -55.8229) (-126.2285, -55.8076) (-125.9802, -55.795) knots 0 0 0 0 1 1 1 1
  spline S718 degree 3 poles (-125.9802, -55.795) (-125.8421, -55.7857) (-125.7039, -55.7765) (-125.5616, -55.7671) knots 0 0 0 0 1 1 1 1
  spline S719 degree 3 poles (-125.5616, -55.7671) (-124.9391, -55.8807) (-124.7328, -56.1471) (-124.3431, -56.6383) knots 0 0 0 0 1 1 1 1
  spline S720 degree 3 poles (-124.3431, -56.6383) (-124.2734, -57.1025) (-124.2495, -57.4702) (-124.2656, -57.9313) knots 0 0 0 0 1 1 1 1
  spline S721 degree 3 poles (-124.2656, -57.9313) (-124.2673, -58.1146) (-124.2673, -58.1146) (-124.269, -58.3016) knots 0 0 0 0 1 1 1 1
  spline S722 degree 3 poles (-124.269, -58.3016) (-124.2734, -58.6899) (-124.2834, -59.0778) (-124.2935, -59.466) knots 0 0 0 0 1 1 1 1
  spline S723 degree 3 poles (-124.2935, -59.466) (-124.2975, -59.7301) (-124.3011, -59.9942) (-124.3043, -60.2582) knots 0 0 0 0 1 1 1 1
  spline S724 degree 3 poles (-124.3043, -60.2582) (-124.3131, -60.9038) (-124.3267, -61.5491) (-124.3431, -62.1946) knots 0 0 0 0 1 1 1 1
  spline S725 degree 3 poles (-124.3431, -62.1946) (-124.0288, -62.1946) (-123.7144, -62.1946) (-123.3906, -62.1946) knots 0 0 0 0 1 1 1 1
  spline S726 degree 3 poles (-123.3906, -62.1946) (-123.3906, -62.4041) (-123.3906, -62.6137) (-123.3906, -62.8296) knots 0 0 0 0 1 1 1 1
  spline S727 degree 3 poles (-123.3906, -62.8296) (-123.7049, -62.8296) (-124.0192, -62.8296) (-124.3431, -62.8296) knots 0 0 0 0 1 1 1 1
  spline S728 degree 3 poles (-124.3431, -62.8296) (-124.3431, -63.6154) (-124.3431, -64.4012) (-124.3431, -65.2108) knots 0 0 0 0 1 1 1 1
  spline S729 degree 3 poles (-126.5656, -77.5933) (-126.8799, -77.5933) (-127.1942, -77.5933) (-127.5181, -77.5933) knots 0 0 0 0 1 1 1 1
  spline S730 degree 3 poles (-127.5181, -77.5933) (-127.5181, -74.6596) (-127.5181, -71.7259) (-127.5181, -68.7033) knots 0 0 0 0 1 1 1 1